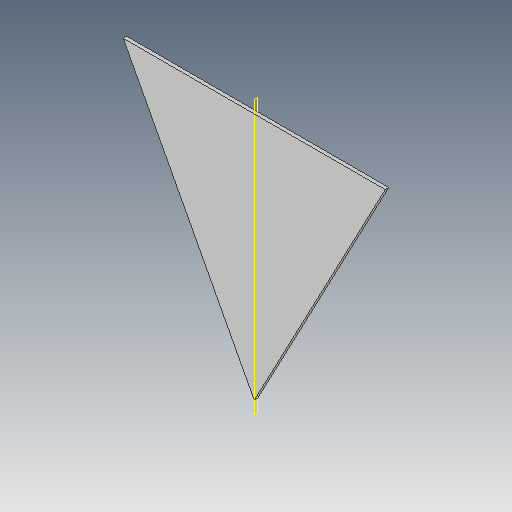
# Autodesk Inventor part: origami03
Saved by Autodesk Inventor 2019.4 (Build 234330000, 330)
## iProperties
Created: 2018-08-06
Part Number: origami03
Material: 一般
Document SubType Name: Modeling
Designer: AzLIer
Density: 1 g/cm^3
Appearance: 既定
Author: AzLIer
Autodesk Inventor part; units mm, degrees
ref_plane "YZ Plane" through (0, 0, 0) normal (1, 0, 0) x (0, 1, 0)
ref_plane "XZ Plane" through (0, 0, 0) normal (0, 1, 0) x (-1, 0, 0)
ref_plane "XY Plane" through (0, 0, 0) normal (0, 0, 1) x (1, 0, 0)
sketch "スケッチ1" plane through (0, 0, 0) normal (0, 0, 1) x (1, 0, 0)
  line L0 (37, -100) -> (-37, -100)
  line L1 (-37, -100) -> (-37, 100)
  line L2 (-37, 100) -> (37, 100)
  line L3 (37, 100) -> (37, -100)
  line L4 (37, -100) -> (-37, 100) construction
  line L5 (-37, -100) -> (37, 100) construction
  line L6 (-37, 0) -> (37, 0) construction
  line L7 (37, 0) -> (0, 30)
  line L8 (0, 30) -> (-37, 0)
  line L9 (-37, 0) -> (0, -30)
  line L10 (0, -30) -> (37, 0)
  line L11 (0, 30) -> (0, -30)
  line L12 (0, 30) -> (-37, 100)
  line L13 (0, 30) -> (37, 100)
  line L14 (0, -30) -> (-37, -100)
  line L15 (0, -30) -> (37, -100)
  point P0 (0, 0)
  point P1 (0, 0)
  point P2 (0, 0)
  dimension "d0" = 74
  dimension "d1" = 200
  dimension "d2" = 60
  constraints: 32 end point, 7 midpoint, 3 parallel, 2 vertical alignment, 1 horizontal, 1 perpendicular, 1 vertical
  measures "d0" distance of L1.end L2.end
  measures "d1" distance of L0.end L1.end
  measures "d2" distance of L7.end L9.end
extrude "押し出し1" add sketch "スケッチ1" along normal blind 1 contours L13 L12 L2
ref_plane "作業平面1" through (0, 30, 0) normal (1, 0, 0) x (0, 0, 1)
